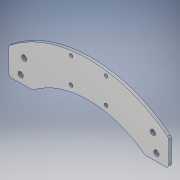
# Autodesk Inventor part: Y Bearing Plate
Saved by Autodesk Inventor 2019 (Build 230136000, 136)
## iProperties
Created: 2018-06-16
Part Number: Y Bearing Plate
Material: Aluminum 6061
Document SubType Name: Modeling
Designer: Richard
Density: 2.7 g/cm^3
Appearance: Aluminum - Flat
Author: Richard
Autodesk Inventor part; units mm, degrees
ref_plane "YZ Plane" through (0, 0, 0) normal (1, 0, 0) x (0, 1, 0)
ref_plane "XZ Plane" through (0, 0, 0) normal (0, 1, 0) x (-1, 0, 0)
ref_plane "XY Plane" through (0, 0, 0) normal (0, 0, 1) x (1, 0, 0)
sketch "Sketch1" plane through (0, 0, 0) normal (0, 0, 1) x (1, 0, 0)
  line L0 (-91.5, -8.5) -> (-64, -8.5)
  line L1 (-91.5, 21.5) -> (-91.5, -8.5)
  line L2 (64, -8.5) -> (91.5, -8.5)
  line L3 (91.5, -8.5) -> (91.5, 21.5)
  arc A0 (64, -8.5) -> (-64, -8.5) centre (0, -90.5909) ccw
  arc A1 (91.5, 21.5) -> (-91.5, 21.5) centre (0, -90.5909) ccw
  circle A2 centre (-77.5, 0) radius 3
  circle A3 centre (77.5, 0) radius 3
  circle A4 centre (-73.5, 18.5) radius 3
  circle A5 centre (73.5, 18.5) radius 3
  line L4 (-20, 18.5) -> (20, 18.5) construction
  line L5 (20, 18.5) -> (20, 47.5) construction
  line L6 (20, 47.5) -> (-20, 47.5) construction
  line L7 (-20, 47.5) -> (-20, 18.5) construction
  line L8 (-20, 18.5) -> (20, 47.5) construction
  line L9 (20, 18.5) -> (-20, 47.5) construction
  circle A6 centre (-20, 47.5) radius 2
  circle A7 centre (20, 47.5) radius 2
  circle A8 centre (20, 18.5) radius 2
  circle A9 centre (-20, 18.5) radius 2
  point P0 (0, 0)
  point P1 (0, 33)
  point P2 (0, 33)
  dimension "d0" = 155
  dimension "d1" = 77.5
  dimension "d2" = 8.5
  dimension "d3" = 27.5
  dimension "d4" = 14
  dimension "d5" = 14
  dimension "d6" = 30
  dimension "d12" = 6
  dimension "d13" = 18.5
  dimension "d14" = 4
  dimension "d15" = 18.5
  dimension "d16" = 4
  dimension "d17" = 40
  dimension "d18" = 29
  dimension "d19" = 4
  dimension "d20" = 22
  constraints: 20 end point, 10 centre point, 8 coincident, 6 equal radius, 4 point on circle, 3 horizontal, 3 horizontal alignment, 3 midpoint, 2 equal length, 2 parallel, 2 perpendicular, 1 collinear, 1 concentric, 1 vertical, 1 vertical alignment
  measures "d0" distance of point (77.5, 0) point (-77.5, 0)
  measures "d1" distance of point (0, 0) point (-77.5, 0)
  measures "d2" distance from line of L2 point (77.5, 0)
  measures "d3" distance of L0.start L0.end
  measures "d4" distance from line of point (-77.5, 0) L1
  measures "d5" distance from line of L3 point (77.5, 0)
  measures "d6" distance of L1.start L0.start
  measures "d12" diameter of A2
  measures "d13" vertical distance of A4.centre point (-77.5, 0)
  measures "d14" horizontal distance of A4.centre A2.centre
  measures "d15" vertical distance of A5.centre point (77.5, 0)
  measures "d16" horizontal distance of A3.centre A5.centre
  measures "d17" distance of L6.end L5.end
  measures "d18" distance of L5.end L4.end
  measures "d19" diameter of A6
  measures "d20" distance edge to line of A0 L0
extrude "Extrusion1" add sketch "Sketch1" along normal mid plane 3.1242
fillet "Fillet1" radius 4 6 edges at (-91.5, -8.5, 0) (-91.5, 21.5, 0) (-64, -8.5, 0) (64, -8.5, 0) (91.5, -8.5, 0) (91.5, 21.5, 0)
equation "\"d1\" = 0.5 * d0"
body "Solid1"
